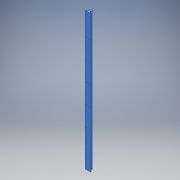
# Autodesk Inventor part: SBR16_EIXO_Y_1
Saved by Autodesk Inventor 2018 (Build 220112000, 112)
## iProperties
Created: 2018-10-09
Part Number: SBR16_EIXO_Y_1
Material: Genérico
Document SubType Name: Modeling
Designer: Georgines
Density: 1 g/cm^3
Appearance: Padrão
Author: Georgines
Autodesk Inventor part; units mm, degrees
ref_plane "YZ Plane" through (0, 0, 0) normal (1, 0, 0) x (0, 1, 0)
ref_plane "XZ Plane" through (0, 0, 0) normal (0, 1, 0) x (-1, 0, 0)
ref_plane "XY Plane" through (0, 0, 0) normal (0, 0, 1) x (1, 0, 0)
sketch "Esboço1" plane through (0, 0, 0) normal (0, 0, 1) x (1, 0, 0)
  arc A0 (4, 2.4377) -> (-4, 2.4377) centre (0, 9.3659) ccw
  line L0 (9.25, -3.9341) -> (9.25, -10.6341)
  line L1 (-9.25, -10.6341) -> (-9.25, -3.9341)
  line L2 (4, -15.6341) -> (-4, -15.6341)
  line L3 (20, -15.6341) -> (-20, -15.6341)
  line L4 (-20, -15.6341) -> (-20, -10.6341)
  line L5 (20, -10.6341) -> (20, -15.6341)
  line L6 (7.6788, -3.9341) -> (9.25, -3.9341)
  line L7 (-9.25, -3.9341) -> (-7.6788, -3.9341)
  line L8 (9.25, -10.6341) -> (20, -10.6341)
  line L9 (-20, -10.6341) -> (-9.25, -10.6341)
  line L10 (-4, 2.4377) -> (-7.6788, -3.9341)
  line L11 (-17.4151, -20.798) -> (-22.4188, -29.4646)
  line L12 (17.4151, -20.798) -> (23.6527, -31.6017)
  line L13 (9.25, -15.6341) -> (4, -15.6341)
  line L14 (0, -15.6341) -> (-9.25, -15.6341)
  line L15 (4, 2.4377) -> (7.6788, -3.9341)
  dimension "d6" = 16
  dimension "d7" = 25
  dimension "d8" = 18.5
  dimension "d9" = 11.7
  dimension "d10" = 8
  dimension "d13" = 5
  dimension "d14" = 40
  constraints: 32 end point, 8 parallel, 3 horizontal, 3 perpendicular, 2 point on circle, 1 centre point, 1 midpoint
  measures "d6" diameter of A0
  measures "d7" distance of A0.centre L14.start
  measures "d8" distance of L13.start L14.end
  measures "d9" distance of L0.start L13.start
  measures "d10" distance of L2.start L2.end
  measures "d13" distance of L3.end L4.end
  measures "d14" distance of L3.start L3.end
extrude "Extrusão1" add sketch "Esboço1" along normal blind 1054
sketch "Esboço3" plane through (-20, -15.6341, 0) normal (0, -1, 0) x (1, 0, 0)
  line L0 (0, 1054) -> (40, 1054) construction
  line L1 (20, 1054) -> (20, 0) construction
  line L2 (20, 1029) -> (5, 1029) construction
  line L3 (5, 1029) -> (20, 1029) construction
  line L4 (20, 1029) -> (35, 1029) construction
  circle A0 centre (5, 1029) radius 2.75
  circle A1 centre (35, 1029) radius 2.75
  line L5 (40, 0) -> (0, 0) construction
  line L6 (35, 1054) -> (35, 0) construction
  line L7 (5, 1054) -> (5, 0) construction
  point P0 (5, 879)
  point P1 (35, 879)
  point P2 (5, 729)
  point P3 (35, 729)
  point P4 (5, 579)
  point P5 (35, 579)
  point P6 (5, 429)
  point P7 (35, 429)
  point P8 (5, 279)
  point P9 (35, 279)
  point P10 (5, 129)
  point P11 (35, 129)
  dimension "d18" = 15
  dimension "d19" = 15
  dimension "d20" = 5.5
  dimension "d21" = 5.5
  dimension "d22" = 25
  dimension "d39" = 150
  constraints: 12 end point, 6 point on line, 2 centre point, 2 coincident, 1 collinear, 1 horizontal, 1 midpoint, 1 vertical
  measures "d18" distance of L2.start L2.end
  measures "d19" distance of L2.start L4.end
  measures "d20" diameter of A0
  measures "d21" diameter of A1
  measures "d22" distance between parallel lines of L0 L2
  measures "d39" distance of A0.centre point (5, 879)
hole "Furo2" at (-15, -15.6341, 279) at (15, -15.6341, 279) at (15, -15.6341, 129) at (-15, -15.6341, 129) at (15, -15.6341, 429) at (-15, -15.6341, 429) at (15, -15.6341, 579) at (-15, -15.6341, 579) at (15, -15.6341, 729) at (-15, -15.6341, 729) at (-15, -15.6341, 879) at (15, -15.6341, 879) at (15, -15.6341, 1029) at (-15, -15.6341, 1029) direction (0, 1, 0) diameter 5.5 end through all
